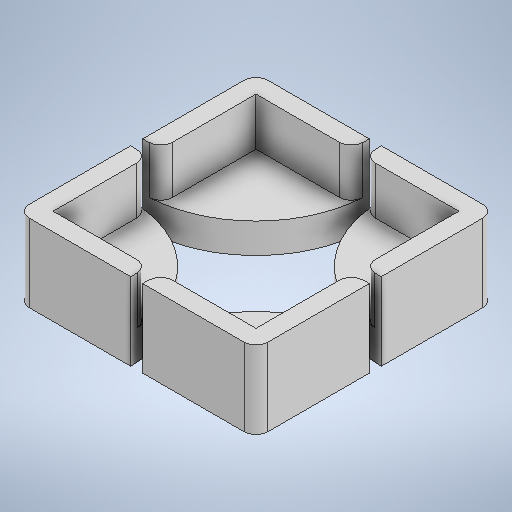
# Autodesk Inventor part: cnc_wood_holder
Saved by Autodesk Inventor 2025.2 (Build 292293000, 293)
## iProperties
Created: 2025-11-29
Part Number: cnc_wood_holder
Material: Generic
Document SubType Name: Modeling
Designer: die02
Density: 1 g/cm^3
Appearance: Default
Author: die02
Autodesk Inventor part; units mm, degrees
ref_plane "YZ Plane" through (0, 0, 0) normal (1, 0, 0) x (0, 1, 0)
ref_plane "XZ Plane" through (0, 0, 0) normal (0, 1, 0) x (-1, 0, 0)
ref_plane "XY Plane" through (0, 0, 0) normal (0, 0, 1) x (1, 0, 0)
sketch "Sketch1" plane through (0, 0, 0) normal (0, 1, 0) x (-1, 0, 0)
  line L0 (-20, 20) -> (20, 20)
  line L1 (20, 20) -> (20, -20)
  line L2 (20, -20) -> (-20, -20)
  line L3 (-20, -20) -> (-20, 20)
  line L4 (-20, 20) -> (20, -20) construction
  line L5 (20, 20) -> (-20, -20) construction
  arc A0 (1, 20) -> (20, 1) centre (20, 20) ccw
  line L6 (20, 20) -> (1, 20) construction
  line L7 (20, 20) -> (20, 1) construction
  arc A1 (-1, -20) -> (-20, -1) centre (-20, -20) ccw
  arc A2 (-20, 1) -> (-1, 20) centre (-20, 20) ccw
  arc A3 (20, -1) -> (1, -20) centre (20, -20) ccw
  point P0 (0, 0)
  point P1 (-1, -20)
  point P2 (-20, -1)
  point P3 (20, -1)
  point P4 (1, -20)
  point P5 (-20, 1)
  point P6 (-1, 20)
  point P7 (1, 20)
  dimension "d0" = 40
  dimension "d1" = 40
  dimension "d2" = 90
  dimension "d3" = 1
  dimension "d6" = 90
  constraints: 16 end point, 8 point on circle, 4 centre point, 3 symmetric about line, 2 midpoint, 2 parallel, 1 coincident, 1 horizontal, 1 perpendicular, 1 point on line, 10 other
  measures "d0" distance of L0.end L1.end
  measures "d1" distance of L1.end L2.end
  measures "d2" angle of L6 L7
  measures "d3" vertical distance of point (0, 0) L7.end
extrude "Extrusion1" add sketch "Sketch1" along normal blind 5 contours L0 A2 L3 | L0 L1 A0 | A1 L2 L3 | L1 L2 A3
sketch "Sketch2" plane through (0, 5, 0) normal (0, 1, 0) x (1, 0, 0)
  line L0 (-20, -1) -> (-20, -20) projected
  line L1 (20, 1) -> (20, 20) projected
  line L2 (-20, 20) -> (-20, -20)
  arc A0 (-1, -20) -> (-20, -1) centre (-20, -20) ccw projected
  arc A1 (-1, -20) -> (-20, -1) centre (-20, -20) ccw
  arc A2 (20, -1) -> (1, -20) centre (20, -20) ccw
  arc A3 (1, 20) -> (20, 1) centre (20, 20) ccw
  arc A4 (-20, 1) -> (-1, 20) centre (-20, 20) ccw
  line L3 (17, -17) -> (1.2383, -17)
  line L4 (-1.2383, -17) -> (-17, -17)
  line L5 (-20, -20) -> (-1, -20)
  line L6 (1, -20) -> (20, -20)
  line L7 (-17, -17) -> (-17, -1.2383)
  line L8 (-17, 1.2383) -> (-17, 17)
  line L9 (-17, 17) -> (-1.2383, 17)
  line L10 (1.2383, 17) -> (17, 17)
  line L11 (20, 20) -> (1, 20)
  line L12 (-1, 20) -> (-20, 20)
  line L13 (17, 17) -> (17, 1.2383)
  line L14 (17, -1.2383) -> (17, -17)
  line L15 (20, -20) -> (20, -1)
  line L16 (20, 1) -> (20, 20)
  point P0 (0, 0)
  point P1 (-20, 1)
  dimension "d13" = 360
  constraints: 30 end point, 16 point on circle, 14 parallel, 8 perpendicular, 4 centre point, 2 horizontal, 1 coincident, 17 other
extrude "Extrusion2" add sketch "Sketch2" along normal blind 8 contours A0 L7 L4 L5 L0 | L2 L12 A4 L9 L8 | A3 L13 L10 L11 L1 | L15 L6 A2 L3 L14
fillet "Fillet1" radius 2 4 edges at (-17, 9, 1.2383) (-17, 9, -1.2383) (-1.2383, 9, 17) (-1.2383, 9, -17)
fillet "Fillet2" radius 2 2 edges at (1.2383, 9, -17) (17, 9, -1.2383)
fillet "Fillet3" radius 2 2 edges at (1.2383, 9, 17) (17, 9, 1.2383)
fillet "Fillet4" radius 2 3 edges at (-20, 6.5, 20) (20, 6.5, 20) (-20, 6.5, -20)
fillet "Fillet5" radius 2 1 edges at (20, 6.5, -20)
body "Solid1"
